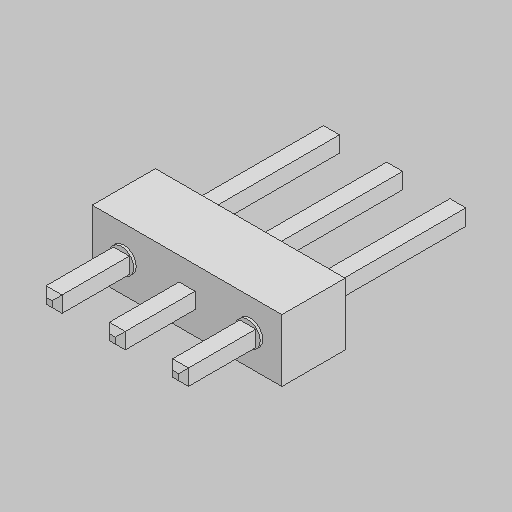
# Autodesk Inventor part: Male_Pin_1x3
Saved by Autodesk Inventor 2023.5 (Build 275446000, 446)
## iProperties
Created: 2024-02-02
Part Number: Male_Pin_1x3
Material: Generic
Document SubType Name: Modeling
Designer: Paul
Density: 1 g/cm^3
Appearance: Default
Author: Paul
Autodesk Inventor part; units mm, degrees
ref_plane "YZ Plane" through (0, 0, 0) normal (1, 0, 0) x (0, 1, 0)
ref_plane "XZ Plane" through (0, 0, 0) normal (0, 1, 0) x (-1, 0, 0)
ref_plane "XY Plane" through (0, 0, 0) normal (0, 0, 1) x (1, 0, 0)
sketch "Sketch1" plane through (0, 0, 0) normal (0, 0, 1) x (1, 0, 0)
  line L0 (0, 0) -> (7.62, 0)
  line L1 (7.62, 0) -> (7.62, 2.5)
  line L2 (7.62, 2.5) -> (0, 2.5)
  line L3 (0, 2.5) -> (0, 0)
  dimension "d0" = 7.62
  dimension "d1" = 2.5
  constraints: 8 end point, 2 parallel, 1 horizontal, 1 perpendicular
  measures "d0" distance of L1.end L2.end
  measures "d1" distance of L0.end L1.end
extrude "Extrusion1" add sketch "Sketch1" along normal blind 2.54
sketch "Sketch2" plane through (0, 0, 2.54) normal (0, 0, 1) x (1, 0, 0)
  line L0 (0.95, 1.57) -> (1.59, 1.57)
  line L1 (1.59, 1.57) -> (1.59, 0.93)
  line L2 (1.59, 0.93) -> (0.95, 0.93)
  line L3 (0.95, 0.93) -> (0.95, 1.57)
  line L4 (3.49, 1.57) -> (4.13, 1.57)
  line L5 (4.13, 1.57) -> (4.13, 0.93)
  line L6 (4.13, 0.93) -> (3.49, 0.93)
  line L7 (3.49, 0.93) -> (3.49, 1.57)
  line L8 (6.03, 1.57) -> (6.67, 1.57)
  line L9 (6.67, 1.57) -> (6.67, 0.93)
  line L10 (6.67, 0.93) -> (6.03, 0.93)
  line L11 (6.03, 0.93) -> (6.03, 1.57)
  line L12 (7.62, 2.5) -> (0, 2.5) projected
  line L13 (0, 2.5) -> (0, 0) projected
  dimension "d4" = 0.64
  dimension "d5" = 0.64
  dimension "d6" = 0.64
  dimension "d7" = 0.64
  dimension "d8" = 2.54
  dimension "d9" = 2.54
  dimension "d10" = 0.93
  dimension "d11" = 0.95
  constraints: 24 end point, 6 parallel, 4 point on line, 3 horizontal, 3 perpendicular
  measures "d4" distance of L0.start L0.end
  measures "d5" distance of L2.end L0.start
  measures "d6" distance of L4.start L4.end
  measures "d7" distance of L8.start L8.end
  measures "d8" distance between parallel lines of L5 L1
  measures "d9" distance between parallel lines of L5 L9
  measures "d10" distance between parallel lines of L12 L0
  measures "d11" distance between parallel lines of L13 L3
extrude "Extrusion2" add sketch "Sketch2" along normal blind 3
sketch "Sketch3" plane through (0, 0, 0) normal (0, 0, -1) x (-1, 0, 0)
  line L0 (-6.03, 0.93) -> (-6.67, 0.93) projected
  line L1 (-6.67, 0.93) -> (-6.67, 1.57) projected
  line L2 (-6.67, 1.57) -> (-6.03, 1.57) projected
  line L3 (-6.03, 1.57) -> (-6.03, 0.93) projected
  line L4 (-3.49, 0.93) -> (-4.13, 0.93) projected
  line L5 (-4.13, 0.93) -> (-4.13, 1.57) projected
  line L6 (-4.13, 1.57) -> (-3.49, 1.57) projected
  line L7 (-3.49, 1.57) -> (-3.49, 0.93) projected
  line L8 (-0.95, 0.93) -> (-1.59, 0.93) projected
  line L9 (-1.59, 0.93) -> (-1.59, 1.57) projected
  line L10 (-1.59, 1.57) -> (-0.95, 1.57) projected
  line L11 (-0.95, 1.57) -> (-0.95, 0.93) projected
  point P0 (0, 0)
extrude "Extrusion3" add sketch "Sketch3" along normal blind 6
chamfer "Chamfer1" distance 0.2 angle 45 24 edges at (1.27, 1.57, -6) (1.59, 1.25, -6) (1.27, 0.93, -6) (0.95, 1.25, -6) (3.81, 1.57, -6) (4.13, 1.25, -6) (3.81, 0.93, -6) (3.49, 1.25, -6) (6.03, 1.25, -6) (6.35, 1.57, -6) (6.67, 1.25, -6) (6.35, 0.93, -6) (6.67, 1.25, 5.54) (6.35, 1.57, 5.54) (6.03, 1.25, 5.54) (6.35, 0.93, 5.54) (4.13, 1.25, 5.54) (3.81, 0.93, 5.54) (3.49, 1.25, 5.54) (3.81, 1.57, 5.54) (1.59, 1.25, 5.54) (1.27, 0.93, 5.54) (0.95, 1.25, 5.54) (1.27, 1.57, 5.54)
sketch "Sketch4" plane through (0, 0, 2.54) normal (0, 0, 1) x (1, 0, 0)
  circle A0 centre (6.35, 1.25) radius 0.5
  circle A1 centre (1.27, 1.25) radius 0.5
  line L0 (0, 2.5) -> (0, 0) projected
  line L1 (0, 0) -> (7.62, 0) projected
  line L2 (7.62, 0) -> (7.62, 2.5) projected
  dimension "d21" = 1
  dimension "d22" = 1.27
  dimension "d23" = 1.25
  dimension "d24" = 1.25
  dimension "d25" = 1.27
  constraints: 2 centre point, 1 equal radius
  measures "d21" diameter of A1
  measures "d22" distance from line of A1.centre L0
  measures "d23" distance from line of L1 A1.centre
  measures "d24" distance from line of L1 A0.centre
  measures "d25" distance from line of L2 A0.centre
extrude "Extrusion4" add sketch "Sketch4" along normal blind 0.1
equation "\"d5\" = d4"
equation "\"d6\" = d4"
equation "\"d7\" = d4"
equation "\"d9\" = d8"
equation "\"d24\" = d23"
equation "\"d25\" = d22"
body "Solid1"
